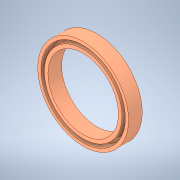
# Autodesk Inventor part: 20_cube_lens_holder_clamp NEW
Saved by Autodesk Inventor 2022 (Build 260153000, 153)
## iProperties
Created: 2020-10-13
Part Number: 20_cube_lens_holder_clamp NEW
Material: Generisch
Document SubType Name: Modeling
Designer: UC2
Density: 1 g/cm^3
Appearance: Vorgabe
Author: UC2
Autodesk Inventor part; units mm, degrees
ref_plane "YZ Plane" through (0, 0, 0) normal (1, 0, 0) x (0, 1, 0)
ref_plane "XZ Plane" through (0, 0, 0) normal (0, 1, 0) x (-1, 0, 0)
ref_plane "XY Plane" through (0, 0, 0) normal (0, 0, 1) x (1, 0, 0)
sketch "Skizze1" plane through (0, 0, 0) normal (0, 0, 1) x (1, 0, 0)
  circle A0 centre (0, 0) radius 11.6
  circle A1 centre (0, 0) radius 14.95
  dimension "d0" = 29.9
  dimension "d1" = 23.2
  dimension "d2" = 3.35
  constraints: 2 centre point, 2 coincident
  measures "d0" diameter of A1
  measures "d1" diameter of A0
  measures "d2" radial gap between concentric circles of A1 A0
extrude "Extrusion1" add sketch "Skizze1" along normal blind 4.5
sketch "Skizze2" plane through (0, 0, 4.5) normal (0, 0, 1) x (1, 0, 0)
  circle A0 centre (0, 0) radius 12.8
  circle A1 centre (0, 0) radius 13.9
  circle A2 centre (0, 0) radius 11.6 projected
  circle A3 centre (0, 0) radius 14.95 projected
  dimension "d5" = 25.6
  dimension "d6" = 27.8
  dimension "d7" = 1.1
  dimension "d8" = 1.2
  dimension "d9" = 1.05
  constraints: 2 centre point, 2 coincident
  measures "d5" diameter of A0
  measures "d6" diameter of A1
  measures "d7" radial gap between concentric circles of A1 A0
  measures "d8" radial gap between concentric circles of A0 A2
  measures "d9" radial gap between concentric circles of A3 A1
extrude "Extrusion2" cut sketch "Skizze2" against normal blind 3 contours A1
